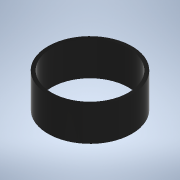
# Autodesk Inventor part: CAN - LOWER
Saved by Autodesk Inventor 2022 (Build 260153000, 153)
## iProperties
Created: 2022-07-25
Part Number: CAN - LOWER
Material: Stainless Steel
Document SubType Name: Modeling
Designer: Nathan Cai
Density: 8 g/cm^3
Appearance: Smooth - Black
Author: Nathan Cai
Autodesk Inventor part; units mm, degrees
ref_plane "YZ Plane" through (0, 0, 0) normal (1, 0, 0) x (0, 1, 0)
ref_plane "XZ Plane" through (0, 0, 0) normal (0, 1, 0) x (-1, 0, 0)
ref_plane "XY Plane" through (0, 0, 0) normal (0, 0, 1) x (1, 0, 0)
sketch "Sketch1" plane through (0, 0, 0) normal (0, 1, 0) x (-1, 0, 0)
  circle A0 centre (0, 0) radius 21.25
  circle A1 centre (0, 0) radius 19.5
  dimension "d0" = 42.5
  dimension "d1" = 1.75
  constraints: 2 centre point, 1 coincident
  measures "d0" diameter of A0
  measures "d1" radial gap between concentric circles of A0 A1
extrude "Extrusion1" add sketch "Sketch1" along normal blind 17.25
body "Solid1"
